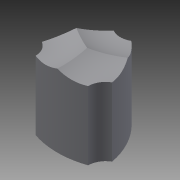
# Autodesk Inventor part: VOLUME
Saved by Autodesk Inventor 2013 (Build 170138000, 138)
## iProperties
Created: 2013-12-08
Part Number: VOLUME
Material: Generic
Document SubType Name: Modeling
Designer: employee
Density: 1 g/cm^3
Author: employee
Autodesk Inventor part; units mm, degrees
ref_plane "YZ Plane" through (0, 0, 0) normal (1, 0, 0) x (0, 1, 0)
ref_plane "XZ Plane" through (0, 0, 0) normal (0, 1, 0) x (-1, 0, 0)
ref_plane "XY Plane" through (0, 0, 0) normal (0, 0, 1) x (1, 0, 0)
sketch "Sketch1" plane through (0, 0, 0) normal (0, 0, 1) x (1, 0, 0)
  line L0 (-150, -86.6025) -> (0, 173.2051) construction
  line L1 (0, 173.2051) -> (150, -86.6025) construction
  line L2 (150, -86.6025) -> (-150, -86.6025) construction
  arc A0 (120.0417, -34.617) -> (30.0416, 121.2676) centre (-150, -86.6025) ccw
  arc A1 (-90, -86.6506) -> (-120.0417, -34.617) centre (-150, -86.6025) ccw
  arc A2 (120.0417, -34.617) -> (90, -86.6506) centre (150, -86.6025) ccw
  arc A3 (-30.0416, 121.2676) -> (30.0416, 121.2676) centre (0, 173.2051) ccw
  arc A4 (-30.0416, 121.2676) -> (-120.0417, -34.617) centre (150, -86.6025) ccw
  arc A5 (-90, -86.6506) -> (90, -86.6506) centre (0, 173.2051) ccw
  point P0 (0, 0)
  point P1 (0, 0)
  dimension "d0" = 300
  dimension "d2" = 120
  dimension "d3" = 275
  constraints: 12 point on circle, 7 coincident, 6 centre point, 6 end point, 4 equal radius, 1 horizontal, 7 other
  measures "d0" distance of L1.end L0.start
  measures "d2" diameter of A1
  measures "d3" radius of A0
extrude "Extrusion1" add sketch "Sketch1" along normal blind 260
sketch "Sketch2" plane through (0, 0, 0) normal (1, 0, 0) x (0, 1, 0)
  line L0 (113.2051, 260) -> (113.2051, 0) projected
  line L1 (113.2051, 0) -> (-101.7949, 0) projected
  line L2 (-101.7949, 0) -> (-101.7949, 260) projected
  line L3 (-101.7949, 260) -> (113.2051, 260) projected
  line L4 (0, 0) -> (0, 260)
  arc A0 (173.2051, 619.634) -> (173.2051, 248.8241) centre (98.2051, 434.2291) ccw
  line L5 (113.2051, 260) -> (121.2676, 260) projected
  line L6 (173.2051, -124.8458) -> (173.2051, 749.0749) projected
  line L7 (173.2051, 619.634) -> (173.2051, 248.8241)
  dimension "d6" = 75
  dimension "d7" = 400
  constraints: 4 end point, 3 point on circle, 3 point on line, 1 centre point, 1 perpendicular
  measures "d6" distance from line of L6 A0.centre
  measures "d7" diameter of A0
revolve "Revolution1" cut sketch "Sketch2" angle 360 about axis through (0, 173.2051, 0) along (0, 0, 1) contours L3 A0 L6 L0 | L0 A0 L3
pattern_circular "Circular Pattern1" count 3 over 360 about axis through (0, 0, -10) along (0, 0, 1) of "Revolution1"
body "Solid1"
